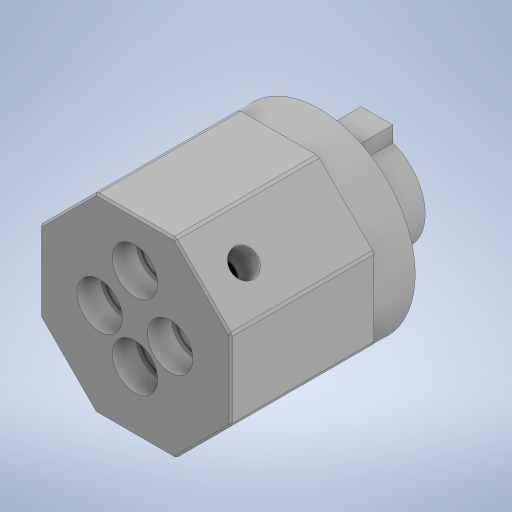
# Autodesk Inventor part: spool_main_drive
Saved by Autodesk Inventor 2023.4 (Build 274418000, 418)
## iProperties
Created: 2023-11-23
Part Number: spool_main_drive
Material: Generic
Document SubType Name: Modeling
Designer: aaron
Density: 1 g/cm^3
Appearance: Default
Author: aaron
Autodesk Inventor part; units mm, degrees
ref_plane "YZ Plane" through (0, 0, 0) normal (1, 0, 0) x (0, 1, 0)
ref_plane "XZ Plane" through (0, 0, 0) normal (0, 1, 0) x (-1, 0, 0)
ref_plane "XY Plane" through (0, 0, 0) normal (0, 0, 1) x (1, 0, 0)
sketch "Sketch1" plane through (0, 0, 0) normal (0, 0, 1) x (1, 0, 0)
  circle A0 centre (0, 0) radius 7.575
  line L0 (-2.5, 9.575) -> (2.5, 9.575)
  line L1 (2.5, 9.575) -> (2.5, 4.3055)
  line L2 (2.5, 4.3055) -> (-2.5, 4.3055)
  line L3 (-2.5, 4.3055) -> (-2.5, 9.575)
  point P0 (-2.5, 7.1506)
  point P1 (2.5, 7.1506)
  dimension "d0" = 15.15
  dimension "d1" = 2.5
  dimension "d2" = 5
  dimension "d3" = 2
  constraints: 8 end point, 2 parallel, 1 centre point, 1 coincident, 1 horizontal, 1 perpendicular
  measures "d0" diameter of A0
  measures "d1" distance from line of L1 point (0, 0)
  measures "d2" distance of L0.start L0.end
  measures "d3" distance edge to line of A0 L0
extrude "Extrusion1" add sketch "Sketch1" along normal blind 10
sketch "Sketch2" plane through (0, 0, 10) normal (0, 0, 1) x (1, 0, 0)
  circle A0 centre (0, 0) radius 15
  dimension "d6" = 30
  constraints: 1 centre point, 1 coincident
  measures "d6" diameter of A0
extrude "Extrusion2" add sketch "Sketch2" along normal blind 5.5
sketch "Sketch3" plane through (0, 0, 10) normal (0, 0, -1) x (-1, 0, 0)
  circle A0 centre (0, 0) radius 13.5
  circle A1 centre (0, 0) radius 15 projected
  dimension "d9" = 27
  constraints: 1 centre point, 1 coincident
  measures "d9" diameter of A0
extrude "Extrusion3" add sketch "Sketch3" along normal blind 1
chamfer "Chamfer1" distance 1 angle 45 1 edges at (13.5, 0, 10)
sketch "Sketch4" plane through (0, 0, 0) normal (0, 0, -1) x (-1, 0, 0)
  arc A0 (7.4833, 0.5) -> (7.4833, -0.5) centre (0, 0) ccw
  circle A1 centre (0, 0) radius 5.55
  circle A2 centre (0, 7.5) radius 2
  arc A3 (-2.5, 7.1506) -> (2.5, 7.1506) centre (0, 0) ccw projected
  line L0 (0, 0) -> (16.7608, 0)
  arc A4 (7.4865, 0.5) -> (7.4865, -0.5) centre (5.55, 0) ccw
  line L1 (0, 0.5) -> (5.5274, 0.5)
  line L2 (7.4833, 0.5) -> (7.5585, 0.5)
  line L3 (0, -0.5) -> (5.5274, -0.5)
  line L4 (7.4833, -0.5) -> (7.5585, -0.5)
  arc A5 (7.5585, -0.5) -> (7.5585, 0.5) centre (0, 0) ccw
  arc A6 (1.9908, 7.3087) -> (-1.9908, 7.3087) centre (0, 0) ccw
  arc A7 (-0.5, 7.4865) -> (0.5, 7.4865) centre (0, 5.55) ccw
  line L5 (-0.5, 7.4833) -> (-0.5, 7.5585)
  arc A8 (0.5, 7.5585) -> (-0.5, 7.5585) centre (0, 0) ccw
  line L6 (0.5, 7.4833) -> (0.5, 7.5585)
  arc A9 (-7.4865, -0.5) -> (-7.4865, 0.5) centre (-5.55, 0) ccw
  line L7 (-7.4833, -0.5) -> (-7.5585, -0.5)
  arc A10 (-7.5585, 0.5) -> (-7.5585, -0.5) centre (0, 0) ccw
  line L8 (-7.4833, 0.5) -> (-7.5585, 0.5)
  arc A11 (0.5, -7.4865) -> (-0.5, -7.4865) centre (0, -5.55) ccw
  line L9 (0.5, -7.4833) -> (0.5, -7.5585)
  arc A12 (-0.5, -7.5585) -> (0.5, -7.5585) centre (0, 0) ccw
  line L10 (-0.5, -7.4833) -> (-0.5, -7.5585)
  point P0 (-7.4822, 0.5163)
  point P1 (-7.4822, -0.5163)
  point P2 (0.5163, -7.4822)
  point P3 (-0.5163, -7.4822)
  point P4 (-0.5, -7.5585)
  point P5 (7.4822, -0.5163)
  point P6 (7.4822, 0.5163)
  dimension "d15" = 4
  dimension "d16" = 15
  dimension "d17" = 4
  dimension "d18" = 11.1
  dimension "d23" = 360
  constraints: 28 point on circle, 22 end point, 12 centre point, 9 point on line, 4 parallel, 3 coincident, 1 horizontal, 49 other
  measures "d15" diameter of A2
  measures "d16" diameter of A0
  measures "d17" diameter of A4
  measures "d18" diameter of A1
extrude "Extrusion4" cut sketch "Sketch4" against normal through all contours A0 A7 A2 A1 | L6 A7 A0 | A0 L5 A6 L6 | A0 A7 L5 | A7 L6 A6 A2 A0 | A0 A2 A7 | A7 A2 A0 | A0 A2 A6 L5 A7 | A6 A2 | A0 L2 A3 L0 A1 A4 | A2 A1 | A9 A1 A0 | A1 L1 A4 | A0 L7 A3 L8 | A9 A1 | A1 L0 A4 L1 | A3 L4 A0 A4 A1 L0 | A1 L3 A4 L0 | A11 A1 | A1 A11 A0 | A1 A4 L3 | L10 A0 L9 A3
sketch "Sketch5" plane through (0, 0, 15.5) normal (0, 0, 1) x (1, 0, 0)
  circle A0 centre (0, 7.5) radius 2 projected
  arc A1 (7.4822, 0.5163) -> (7.4822, -0.5163) centre (5.55, 0) ccw projected
  circle A2 centre (5.55, 0) radius 2
  arc A3 (0.5163, -7.4822) -> (-0.5163, -7.4822) centre (0, -5.55) ccw projected
  circle A4 centre (0, -5.55) radius 2
  arc A5 (-7.4822, -0.5163) -> (-7.4822, 0.5163) centre (-5.55, 0) ccw projected
  circle A6 centre (-5.55, 0) radius 2
  line L0 (0, 0) -> (0, 25.3471)
  line L1 (-2.1083, 23.3215) -> (21.8582, -0.645)
  circle A7 centre (0, 0) radius 15 projected
  line L2 (-17.9816, 15) -> (15.9121, 15)
  line L3 (-23.3215, -2.1083) -> (0.645, 21.8582)
  line L4 (-15, -17.9816) -> (-15, 15.9121)
  line L5 (2.1083, -23.3215) -> (-21.8582, 0.645)
  line L6 (17.9816, -15) -> (-15.9121, -15)
  line L7 (23.3215, 2.1083) -> (-0.645, -21.8582)
  line L8 (15, 17.9816) -> (15, -15.9121)
  point P0 (-7.4822, -0.5163)
  point P1 (-7.4822, 0.5163)
  point P2 (7.4822, -0.5163)
  point P3 (7.4822, 0.5163)
  point P4 (0.5163, -7.4822)
  point P5 (-0.5163, -7.4822)
  point P6 (-6.2132, 15)
  point P7 (-15, 6.2132)
  point P8 (-15, -6.2132)
  point P9 (-6.2132, -15)
  point P10 (6.2132, -15)
  point P11 (15, -6.2132)
  point P12 (15, 6.2132)
  point P13 (6.2132, 15)
  dimension "d27" = 45
  dimension "d30" = 360
  constraints: 18 end point, 3 centre point, 3 coincident, 1 tangent, 1 vertical, 25 other
  measures "d27" angle of L1 L0
extrude "Extrusion5" add sketch "Sketch5" along normal blind 22.55 contours L2 L1 A7 | A7 | A7 L3 L2 | L1 L8 A7 | A7 L4 L3 | L8 L7 A7 | A7 L5 L4 | L7 L6 A7 | A7 L6 L5
sketch "Sketch6" plane through (0, 0, 38.05) normal (0, 0, 1) x (1, 0, 0)
  circle A0 centre (0, 7.5) radius 2 projected
  circle A1 centre (0, 7.5) radius 3.55
  arc A2 (7.4822, 0.5163) -> (7.4822, -0.5163) centre (5.55, 0) ccw projected
  circle A3 centre (5.55, 0) radius 3.55
  arc A4 (0.5163, -7.4822) -> (-0.5163, -7.4822) centre (0, -5.55) ccw projected
  circle A5 centre (0, -5.55) radius 3.55
  arc A6 (-7.4822, -0.5163) -> (-7.4822, 0.5163) centre (-5.55, 0) ccw projected
  circle A7 centre (-5.55, 0) radius 3.55
  point P0 (0, 0)
  dimension "d34" = 7.1
  dimension "d35" = 7.1
  dimension "d36" = 7.1
  dimension "d37" = 7.1
  constraints: 4 centre point, 4 coincident
  measures "d34" diameter of A1
  measures "d35" diameter of A3
  measures "d36" diameter of A5
  measures "d37" diameter of A7
extrude "Extrusion6" cut sketch "Sketch6" against normal blind 4.1
chamfer "Chamfer2" distance 0.3 angle 45 16 edges at (-6.2132, 15, 26.775) (6.2132, 15, 26.775) (15, 6.2132, 26.775) (15, -6.2132, 26.775) (6.2132, -15, 26.775) (-6.2132, -15, 26.775) (0, -15, 38.05) (10.6066, -10.6066, 38.05) (15, 0, 38.05) (10.6066, 10.6066, 38.05) (0, 15, 38.05) (-10.6066, 10.6066, 38.05) (-15, 0, 38.05) (-10.6066, -10.6066, 38.05) (-15, -6.2132, 26.775) (-15, 6.2132, 26.775)
chamfer "Chamfer3" distance 1 angle 45 7 edges at (0, -3.55, 33.95) (0, -7.55, 33.95) (-3.55, 0, 33.95) (-7.55, 0, 33.95) (-2, 7.5, 33.95) (3.55, 0, 33.95) (7.55, 0, 33.95)
chamfer "Chamfer4" distance 0.3 angle 45 4 edges at (-9.1, 0, 33.95) (-3.55, 7.5, 33.95) (2, 0, 33.95) (-3.55, -5.55, 33.95)
sketch "Sketch8" plane through (14.7879, 6.4253, 15.5) normal (0.7071068, 0.7071068, 0) x (-0.7071068, 0.7071068, 0)
  circle A0 centre (5.9132, 16.05) radius 2.1
  line L0 (12.0021, 22.55) -> (-0.1757, 22.55) projected
  line L1 (0, 0) -> (0, 22.25) projected
  line L2 (11.8264, 22.25) -> (11.8264, 0) projected
  point P0 (5.9132, -15.5)
  dimension "d49" = 4.2
  dimension "d50" = 6.5
  dimension "d51" = 11.8264
  dimension "d52" = 5.9132
  constraints: 1 centre point
  measures "d49" diameter of A0
  measures "d50" distance from line of L0 A0.centre
  measures "d51" distance between parallel lines of L1 L2
  measures "d52" distance from line of L1 A0.centre
extrude "Extrusion7" cut sketch "Sketch8" against normal blind 5
sketch "Sketch9" plane through (0, 0, 0) normal (0, 0, -1) x (-1, 0, 0)
  circle A0 centre (0, 0) radius 7.575
  line L0 (-2.5, 7.1506) -> (-2.5, 9.575) projected
  line L1 (-2.5, 9.575) -> (2.5, 9.575) projected
  line L2 (2.5, 9.575) -> (2.5, 7.1506) projected
  circle A1 centre (0, 7.5) radius 2 projected
  circle A2 centre (0, 7.5) radius 1.5
  arc A3 (7.4822, 0.5163) -> (7.4822, -0.5163) centre (5.55, 0) ccw projected
  circle A4 centre (5.55, 0) radius 1.5
  circle A5 centre (0, -5.55) radius 2 projected
  circle A6 centre (0, -5.55) radius 1.5
  circle A7 centre (-5.55, 0) radius 2 projected
  circle A8 centre (-5.55, 0) radius 1.5
  dimension "d55" = 3
  dimension "d56" = 3
  dimension "d57" = 3
  dimension "d58" = 3
  constraints: 5 centre point, 5 coincident
  measures "d55" diameter of A2
  measures "d56" diameter of A4
  measures "d57" diameter of A6
  measures "d58" diameter of A8
extrude "Extrusion8" add sketch "Sketch9" against normal blind 30.55 contours A0 A1 | A0 A1 L0 L1 L2 | A1 A0 A2 | A0 A2 A1 | A5 | A7
chamfer "Chamfer5" distance 0.5 angle 45 4 edges at (-2, 7.5, 30.55) (3.6178, -0.5163, 30.55) (-3.6178, 0.5163, 30.55) (-0.5163, -3.6178, 30.55)
equation "\"d1\" = 0.5 * d2"
equation "\"d52\" = 0.5 * d51"
body "Solid1"
